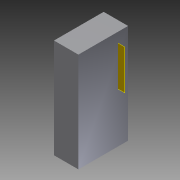
# Autodesk Inventor part: tt
Saved by Autodesk Inventor 2011 SP2 (Build 150309200, 309)
## iProperties
Created: 2012-04-19
Part Number: tt
Document SubType Name: Modeling
Designer: sungwook
Density: 1 g/cm^3
Author: sungwook
Autodesk Inventor part; units mm, degrees
ref_plane "YZ Plane" through (0, 0, 0) normal (1, 0, 0) x (0, 1, 0)
ref_plane "XY Plane" through (0, 0, 0) normal (0, 0, 1) x (1, 0, 0)
sketch "Sketch1" plane through (0, 0, 0) normal (0, 0, 1) x (1, 0, 0)
  point P0 (0, 0)
ref_plane "Work Plane1" through (0, 8.3, 0) normal (0, 1, 0) x (-1, 0, 0)
sketch "Sketch2" plane through (0, 8.3, 0) normal (0, 1, 0) x (-1, 0, 0)
  line L0 (-6.6628, 15) -> (5.6244, 15)
  line L1 (5.6244, 15) -> (5.6244, -35)
  line L2 (5.6244, -35) -> (-6.6628, -35)
  line L3 (-6.6628, -35) -> (-6.6628, 15)
  point P0 (0, 0)
  dimension "d1" = 50
  dimension "d2" = 15
  constraints: 8 end point, 2 parallel, 1 horizontal, 1 perpendicular
  measures "d1" distance between parallel lines of L2 L0
  measures "d2" distance from line of point (0, 0) L0
extrude "Extrusion1" add sketch "Sketch2" along normal blind 5 and the other way blind 20
body "Solid1"
